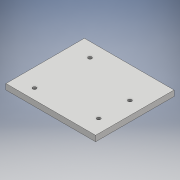
# Autodesk Inventor part: UNO-Mounting-Holes
Saved by Autodesk Inventor 2018 (Build 220112000, 112)
## iProperties
Created: 2022-01-10
Part Number: UNO-Mounting-Holes
Material: Generic
Document SubType Name: Modeling
Designer: Stewart Alexander
Density: 1 g/cm^3
Appearance: Default
Author: Stewart Alexander
Autodesk Inventor part; units mm, degrees
ref_plane "YZ Plane" through (0, 0, 0) normal (1, 0, 0) x (0, 1, 0)
ref_plane "XZ Plane" through (0, 0, 0) normal (0, 1, 0) x (-1, 0, 0)
ref_plane "XY Plane" through (0, 0, 0) normal (0, 0, 1) x (1, 0, 0)
sketch "Arduino Uno" plane through (0, 0, 0) normal (0, 0, 1) x (1, 0, 0)
  line L0 (0, 0) -> (68.6, 0)
  line L1 (68.6, 0) -> (68.6, 53.3)
  line L2 (68.6, 53.3) -> (0, 53.3)
  line L3 (0, 53.3) -> (0, 0)
  circle A0 centre (14, 2.5) radius 1.6
  circle A1 centre (66.1, 7.6) radius 1.6
  circle A2 centre (66.1, 35.5) radius 1.6
  circle A3 centre (15.3, 50.7) radius 1.6
  dimension "d6" = 68.6
  dimension "d7" = 53.3
  dimension "d34" = 3.2
  dimension "d35" = 2.5
  dimension "d36" = 14
  dimension "d37" = 3.2
  dimension "d38" = 66.1
  dimension "d39" = 7.6
  dimension "d40" = 3.2
  dimension "d41" = 35.5
  dimension "d42" = 66.1
  dimension "d43" = 3.2
  dimension "d44" = 15.3
  dimension "d45" = 50.7
  constraints: 8 end point, 4 centre point, 2 parallel, 1 horizontal, 1 perpendicular
  measures "d6" distance of L2.end L1.end
  measures "d7" distance of L0.end L1.end
  measures "d34" diameter of A0
  measures "d35" vertical distance of L0.start A0.centre
  measures "d36" horizontal distance of L0.start A0.centre
  measures "d37" diameter of A1
  measures "d38" horizontal distance of L0.start A1.centre
  measures "d39" vertical distance of L0.start A1.centre
  measures "d40" diameter of A2
  measures "d41" vertical distance of L0.start A2.centre
  measures "d42" horizontal distance of L0.start A2.centre
  measures "d43" diameter of A3
  measures "d44" horizontal distance of L0.start A3.centre
  measures "d45" vertical distance of L0.start A3.centre
sketch "Sketch2" plane through (0, 0, 0) normal (0, 0, 1) x (1, 0, 0)
  line L0 (0, 0) -> (8, 0)
  line L1 (-2.2793, -6.7051) -> (-2.2793, 63.2949)
  line L2 (-2.2793, 63.2949) -> (77.7207, 63.2949)
  line L3 (77.7207, 63.2949) -> (77.7207, -6.7051)
  line L4 (77.7207, -6.7051) -> (-2.2793, -6.7051)
  dimension "d27" = 8
  dimension "d28" = 70
  dimension "d29" = 80
  constraints: 10 end point, 4 perpendicular, 1 horizontal
  measures "d27" distance of L0.end L0.start
  measures "d28" distance of L1.start L1.end
  measures "d29" distance of L1.end L2.end
extrude "Back Plate" add sketch "Sketch2" against normal blind 5
extrude "Uno Mounting Holes" cut sketch "Arduino Uno" against normal through all contours A0 | A1 | A2 | A3
body "Solid1"
